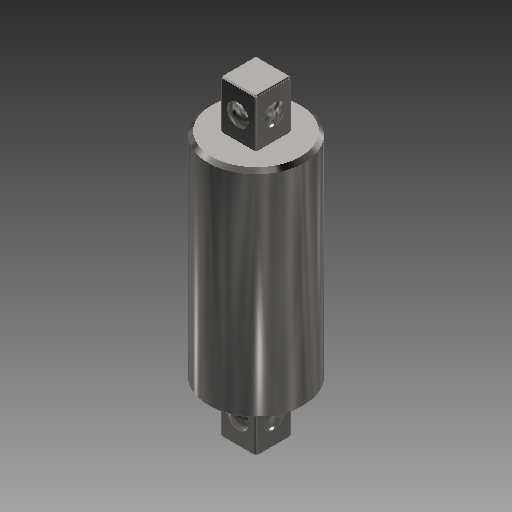
# Autodesk Inventor part: 473-01
Saved by Autodesk Inventor 2019 (Build 230136000, 136)
## iProperties
Company: Autodesk Inc.
Created: 2007-11-28
Part Number: 473-01
Document SubType Name: Modeling
Designer: Autodesk Inc.
Density: 7.85 g/cm^3
Mass: 7.66726 g
Surface Area: 6.3664 cm^2
Volume: 0.976721 cm^3
Material: Steel
Description: MOTOR CONNECTING ROD
Appearance: Steel - Polished
Component Category: Lower Component
Author: Inventor
Autodesk Inventor part; units mm, degrees
ref_plane "YZ Plane" through (0, 0, 0) normal (1, 0, 0) x (0, 1, 0)
ref_plane "XZ Plane" through (0, 0, 0) normal (0, 1, 0) x (-1, 0, 0)
sketch "Sketch1" plane through (0, 0, 0) normal (0, 1, 0) x (-1, 0, 0)
  circle A0 centre (0, 0) radius 4
  dimension "d0" = 8
  constraints: 1 centre point, 1 coincident
  measures "d0" diameter of A0
extrude "Extrusion1" add sketch "Sketch1" against normal mid plane 18
sketch "Sketch2" plane through (0, -9, 0) normal (0, -1, 0) x (1, 0, 0)
  circle A0 centre (0, 0) radius 4 projected
  line L0 (-5.6, 0) -> (5.6, 0) projected
  line L1 (-1.5, -1.5) -> (1.5, -1.5)
  line L2 (1.5, -1.5) -> (1.5, 1.5)
  line L3 (1.5, 1.5) -> (-1.5, 1.5)
  line L4 (-1.5, 1.5) -> (-1.5, -1.5)
  dimension "d3" = 3
  dimension "d4" = 3
  dimension "d5" = 1.5
  dimension "d6" = 1.5
  constraints: 8 end point, 2 parallel, 1 horizontal, 1 perpendicular
  measures "d3" distance of L2.end L3.end
  measures "d4" distance of L3.end L1.start
  measures "d5" distance from line of A0.centre L3
  measures "d6" distance from line of L4 A0.centre
extrude "Extrusion2" add sketch "Sketch2" along normal blind 4 contours L2 L1 L4 L0 | L0 L4 L3 L2
fillet "Fillet1" radius 0.2 8 edges at (1.5, -11, 1.5) (-1.5, -11, 1.5) (1.5, -11, -1.5) (0, -13, -1.5) (-1.5, -13, 0) (0, -13, 1.5) (1.5, -13, 0) (-1.5, -11, -1.5)
sketch "Sketch3" plane through (0, 0, 0) normal (0, 0, 1) x (1, 0, 0)
  line L0 (0, -4.8) -> (0, 0)
  line L1 (2.8, 0) -> (2.8, -4.8)
  arc A0 (-0.35, -2.4) -> (3.15, -2.4) centre (1.4, -2.4) ccw
  line L2 (0, -2.4) -> (2.8, -2.4) construction
  line L3 (-4, -9) -> (-4, 9) projected
  line L4 (-4, 9) -> (4, 9) projected
  line L5 (4, 9) -> (4, -9) projected
  line L6 (4, -9) -> (1.5, -9) projected
  line L7 (1.5, -9) -> (1.5, -12.8) projected
  arc A1 (1.3, -13) -> (1.5, -12.8) centre (1.3, -12.8) ccw projected
  line L8 (1.3, -13) -> (-1.3, -13) projected
  arc A2 (-1.5, -12.8) -> (-1.3, -13) centre (-1.3, -12.8) ccw projected
  line L9 (-1.5, -12.8) -> (-1.5, -9) projected
  line L10 (-1.5, -9) -> (-4, -9) projected
  line L11 (-1.5, -10.9) -> (1.5, -10.9) construction
  arc A3 (-1.75, -10.9) -> (1.75, -10.9) centre (0, -10.9) ccw
  line L12 (1.5, -10.9) -> (2.2631, -10.9) construction
  line L13 (-1.5, -10.9) -> (-1.9787, -10.9) construction
  line L14 (-1.75, -10.9) -> (1.75, -10.9)
  point P0 (1.4, -2.4)
  dimension "d10" = 1.75
  dimension "d11" = 3.5
  constraints: 14 end point, 6 midpoint, 4 point on circle, 4 point on line, 3 collinear, 2 centre point, 1 coincident
  measures "d10" radius of A0
  measures "d11" diameter of A3
revolve "Revolution1" add sketch "Sketch3" angle 360 about axis through (1.5, -10.9, 0) along (1, 0, 0) contours L14 L7 A3 L9 | L9 A3 L14 | L14 A3 L7
mirror "Mirror1" about plane through (0, 0, 0) normal (0, 1, 0) of "Extrusion2", "Revolution1", "Fillet1"
chamfer "Chamfer2" distance 0.3 angle 45 2 edges at (4, -9, 0) (4, 9, 0)
ref_plane "Work Plane2" through (0, 3.5617, 0) normal (0, -1, 0) x (1, 0, 0)
split_face "Split2"
equation "\"d3\" = d4"
equation "\"d5\" = 0.5 * d4"
equation "\"d6\" = 0.5 * d4"
body "Solid1"
